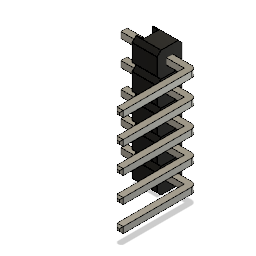
pinsBentAltMale (Autodesk Fusion 360 design; units mm, degrees)
Autodesk Fusion 360 part; units mm, degrees
note: some values were not read from the file. Set by a fixed rule: which sketch regions a step uses.
sketch "Sketch1" plane through (0, 0, 0) normal (0, 1, 0) x (1, 0, 0) in component "Pin"
  line L0 (0, 0) -> (7.239, 0)
  line L1 (7.239, 0) -> (7.239, -7.62)
  line L2 (0, -0.635) -> (0, 0)
  line L3 (7.239, -7.62) -> (6.604, -7.62)
  line L4 (6.604, -7.62) -> (6.604, -0.635)
  line L5 (0, -0.635) -> (6.604, -0.635)
  dimension "d2" = 0.635
  dimension "d3" = 7.239
  dimension "d23" = 7.62
  measures "d3" distance of L0.start
extrude "Extrude1" add sketch "Sketch1" along normal blind 0.635 makes body 1 in component "Pin"
chamfer "Chamfer1" distance 0.1905 angle 45 8 edges at (6.9215, 0.635, 7.62) (6.9215, 0, 7.62) (6.604, 0.3175, 7.62) (7.239, 0.3175, 7.62) (0, 0.3175, 0.635) (0, 0.635, 0.3175) (0, 0.3175, 0) (0, 0, 0.3175) on bodies 1 in component "Pin"
sketch "Sketch1 (2)" plane through (0, 0, 0) normal (0, 1, 0) x (1, 0, 0) in component "Plastic"
  line L0 (0, -0.4445) -> (0, -0.1905)
  line L1 (0, -0.3175) -> (2.921, -0.3175) construction
  line L2 (2.921, -1.0795) -> (2.921, 0.4445)
  line L3 (0.1905, 0) -> (7.239, 0) construction
  line L4 (2.921, 0.4445) -> (2.921, 0.9525) construction
  line L5 (2.921, -1.0795) -> (2.921, -1.5875) construction
  line L6 (2.921, 0.4445) -> (2.286, 0.4445)
  line L7 (2.921, -1.0795) -> (2.286, -1.0795)
  line L8 (2.286, -1.0795) -> (2.286, -1.5875)
  line L9 (2.286, 0.4445) -> (2.286, 0.9525)
  line L10 (2.286, 0.9525) -> (4.826, 0.9525)
  line L11 (4.826, 0.9525) -> (4.826, -1.5875)
  line L12 (2.286, -1.5875) -> (4.826, -1.5875)
  dimension "d7" = 2.921
  dimension "d8" = 1.524
  dimension "d9" = 0.508
  dimension "d11" = 0.635
  dimension "d12" = 2.54
  measures "d7" distance of origin
extrude "Extrude1'" add sketch "Sketch1 (2)" along normal mid plane 2.54 from surface at 0.3175 separate body makes body 2 in component "Plastic"
chamfer "Chamfer1'" distance 0.4 angle 45 4 edges at (3.556, 1.5875, -0.9525) (3.556, -0.9525, -0.9525) (3.556, 1.5875, 1.5875) (3.556, -0.9525, 1.5875) on bodies 2 in component "Plastic"
sketch "Sketch1 (3)" plane through (0, 0, 0) normal (0, 0, 1) x (1, 0, 0)
  line L0 (0, 0.1905) -> (0, 0.4445)
  line L1 (0, 0.3175) -> (0, 14)
fillet "Fillet1" radius 0.5 1 edges at (7.239, 0.3175, 0) on bodies 1 in component "Pin"
other "PathPattern1" in component "Header"
component "Header" placed x (1, 0, 0) y (0, 1, 0) z (0, 0, 1) at (0, 0, 0)
component "Header" placed x (1, 0, 0) y (0, 1, 0) z (0, 0, 1) at (0, 2.54, 0)
component "Header" placed x (1, 0, 0) y (0, 1, 0) z (0, 0, 1) at (0, 5.08, 0)
component "Header" placed x (1, 0, 0) y (0, 1, 0) z (0, 0, 1) at (0, 7.62, 0)
component "Header" placed x (1, 0, 0) y (0, 1, 0) z (0, 0, 1) at (0, 10.16, 0)
component "Pin" placed x (1, 0, 0) y (0, 1, 0) z (0, 0, 1) at (0, 0, 0) in component "Header"
component "Plastic" placed x (1, 0, 0) y (0, 1, 0) z (0, 0, 1) at (0, 0, 0) in component "Header"
equation "pinCount = 5"
equation "d13 = 0.025 in / 2"
equation "d19 = pinCount"
equation "d21 = pinCount"
